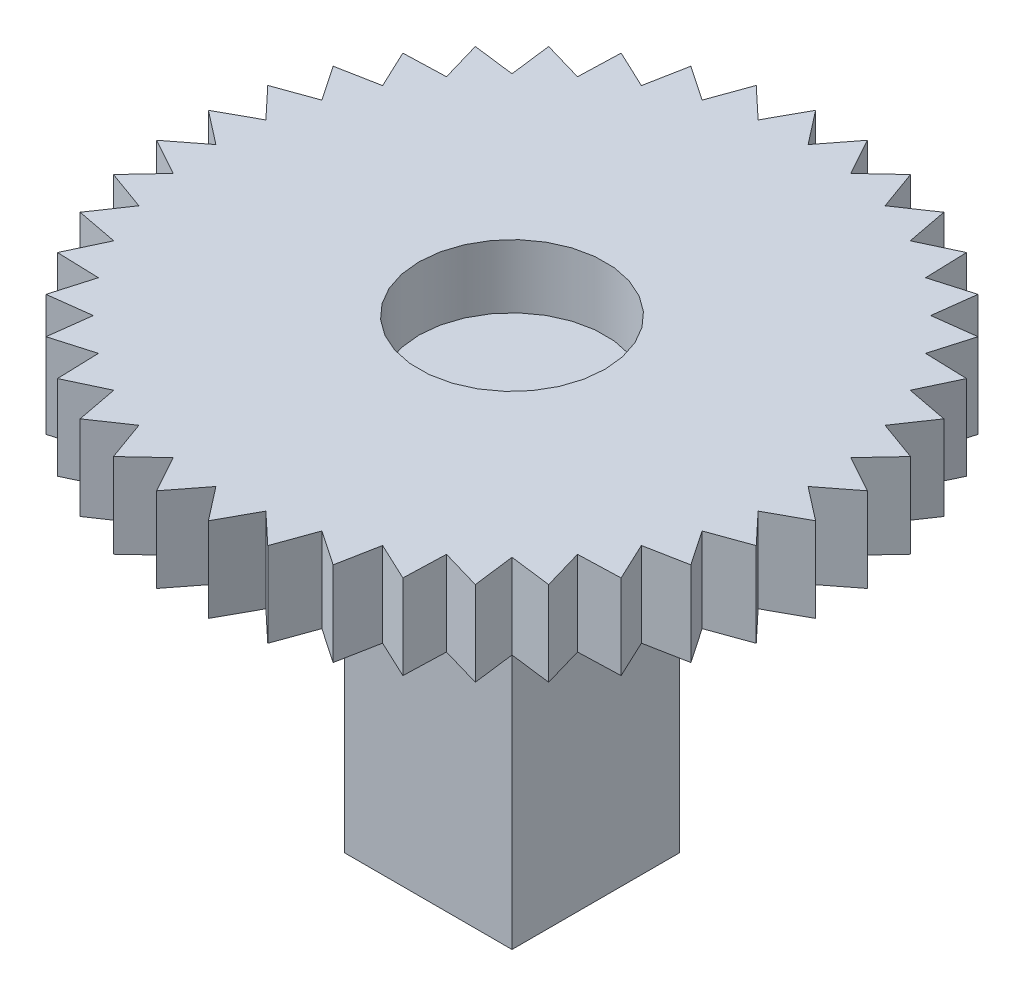
# Autodesk Inventor part: TwoOneGearGtr
Saved by Autodesk Inventor 2015 (Build 190159000, 159)
## iProperties
Created: 2016-04-11
Part Number: TwoOneGearGtr
Material: Generic
Document SubType Name: Modeling
Designer: Hatch
Density: 1 g/cm^3
Appearance: Default
Author: Hatch
Autodesk Inventor part; units mm, degrees
ref_plane "YZ Plane" through (0, 0, 0) normal (1, 0, 0) x (0, 1, 0)
ref_plane "XZ Plane" through (0, 0, 0) normal (0, 1, 0) x (-1, 0, 0)
ref_plane "XY Plane" through (0, 0, 0) normal (0, 0, 1) x (1, 0, 0)
sketch "Sketch1" plane through (0, 0, 0) normal (0, 1, 0) x (-1, 0, 0)
  circle A0 centre (0, 0) radius 35
  dimension "d0" = 70
  constraints: 1 centre point, 1 coincident
  measures "d0" diameter of A0
extrude "Gear Base" add sketch "Sketch1" along normal blind 10
sketch "Sketch2" plane through (0, 10, 0) normal (0, 1, 0) x (1, 0, 0)
  arc A0 (-34.5691, 5.4752) -> (-35, 0) centre (0, 0) ccw
  line L0 (0, 0) -> (-34.5691, 5.4752) construction
  line L1 (0, 0) -> (-35, 0) construction
  line L2 (0, 0) -> (-49.4148, 3.889)
  line L3 (0, 0) -> (49.5676, 0) construction
  line L4 (-35, 0) -> (-38.9501, 3.0654)
  line L5 (-38.9501, 3.0654) -> (-34.5691, 5.4752)
  dimension "d3" = 9
  dimension "d4" = 175.5
  dimension "d5" = 5
  constraints: 12 end point, 2 point on circle, 1 centre point, 1 coincident, 1 equal length, 1 horizontal, 1 point on line
  measures "d3" angle of L0 L1
  measures "d4" angle of L3 L2
  measures "d5" distance of L1.end L4.end
extrude "Gear Tooth" add sketch "Sketch2" against normal blind 10
pattern_circular "Circular Pattern1" count 40 over 360 about axis through (0, 0, 0) along (0, 1, 0) of "Gear Tooth"
sketch "Sketch7" plane through (0, 0, 0) normal (0, -1, 0) x (1, 0, 0)
  line L0 (9.9, 9.9) -> (-9.9, 9.9)
  line L1 (-9.9, 9.9) -> (-9.9, -9.9)
  line L2 (-9.9, -9.9) -> (9.9, -9.9)
  line L3 (9.9, -9.9) -> (9.9, 9.9)
  line L4 (9.9, 9.9) -> (-9.9, -9.9) construction
  line L5 (-9.9, 9.9) -> (9.9, -9.9) construction
  point P0 (0, 0)
  dimension "d23" = 19.8
  dimension "d24" = 19.8
  constraints: 12 end point, 2 midpoint, 2 parallel, 1 horizontal, 1 perpendicular
  measures "d23" distance of L2.end L1.end
  measures "d24" distance of L1.end L0.end
extrude "Extrusion5" add sketch "Sketch7" along normal blind 45
sketch "Sketch8" plane through (0, 0, 0) normal (0, -1, 0) x (1, 0, 0)
  line L0 (-9.9, -9.9) -> (9.9, -9.9)
  line L1 (9.9, -9.9) -> (9.9, 9.9)
  line L2 (9.9, 9.9) -> (-9.9, 9.9)
  line L3 (-9.9, 9.9) -> (-9.9, -9.9)
  line L4 (-9.9, -9.9) -> (9.9, 9.9) construction
  line L5 (9.9, -9.9) -> (-9.9, 9.9) construction
  line L6 (-12.5, -12.5) -> (12.5, -12.5)
  line L7 (12.5, -12.5) -> (12.5, 12.5)
  line L8 (12.5, 12.5) -> (-12.5, 12.5)
  line L9 (-12.5, 12.5) -> (-12.5, -12.5)
  line L10 (-12.5, -12.5) -> (12.5, 12.5) construction
  line L11 (12.5, -12.5) -> (-12.5, 12.5) construction
  point P0 (0, 0)
  dimension "d27" = 25
  dimension "d28" = 25
  constraints: 24 end point, 4 midpoint, 4 parallel, 2 horizontal, 2 perpendicular
  measures "d27" distance of L8.end L7.end
  measures "d28" distance of L7.end L6.end
extrude "Extrusion6" add sketch "Sketch8" along normal blind 10
sketch "Sketch9" plane through (0, 10, 0) normal (0, 1, 0) x (1, 0, 0)
  circle A0 centre (0, 0) radius 11
  dimension "d31" = 22
  constraints: 1 centre point, 1 coincident
  measures "d31" diameter of A0
extrude "Extrusion7" cut sketch "Sketch9" against normal blind 7.5
sketch "Sketch10" plane through (0, -45, 0) normal (0, -1, 0) x (1, 0, 0)
  circle A0 centre (0, 0) radius 11
  dimension "d34" = 22
  constraints: 1 centre point, 1 coincident
  measures "d34" diameter of A0
body "Solid1"
